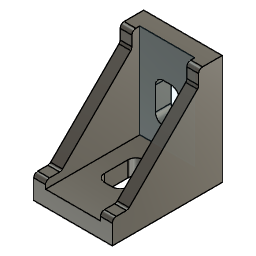
angle_bracket (Autodesk Fusion 360 design; units mm, degrees)
Autodesk Fusion 360 part; units mm, degrees
sketch "Sketch1" plane through (0, 0, 0) normal (1, 0, 0) x (0, 1, 0)
  line L0 (0, 0) -> (28, 0)
  line L1 (28, 0) -> (28, 28)
  line L2 (28, 28) -> (22, 28)
  line L3 (22, 28) -> (22, 24)
  line L4 (0, 0) -> (0, 6)
  line L5 (0, 6) -> (4, 6)
  line L6 (4, 6) -> (22, 24)
  dimension "d1" = 28
  dimension "d2" = 28
  constraint coincident L0.start L4.start
  constraint horizontal L0
  constraint perpendicular L0 L1
  constraint perpendicular L1 L2
  constraint perpendicular L2 L3
  constraint perpendicular L0 L4
  constraint perpendicular L4 L5
  measures "d1" distance of L0.start L0.end
  measures "d2" distance of L0.end L1.end
extrude "Extrude1" add sketch "Sketch1" along normal blind 3
sketch "Sketch2" plane through (3, 0, 0) normal (1, 0, 0) x (0, 1, 0)
  line L0 (0, 0) -> (28, 0)
  line L1 (28, 0) -> (28, 28)
  line L2 (28, 28) -> (22, 28)
  line L3 (22, 28) -> (22, 24)
  line L4 (22, 24) -> (4, 6)
  line L5 (4, 6) -> (0, 6)
  line L6 (0, 6) -> (0, 0)
  line L7 (0, 0) -> (28, 0)
  line L8 (28, 0) -> (28, 4)
  line L9 (24, 4) -> (0, 4)
  line L10 (0, 4) -> (0, 0)
  line L11 (28, 28) -> (24, 28)
  line L12 (24, 28) -> (24, 4)
  line L13 (24, 0) -> (28, 0)
  line L14 (28, 0) -> (28, 28)
  dimension "d5" = 4
  dimension "d6" = 28
  constraint horizontal L7
  constraint vertical L8
  constraint horizontal L9
  constraint vertical L10
  constraint coincident L1 L8.end
  constraint coincident L0.start L6.end
  constraint horizontal L11
  constraint vertical L12
  constraint horizontal L13
  constraint vertical L14
  constraint coincident L1.end L2.start
  measures "d5" distance of L1.end L11.end
  measures "d6" distance of L1.end L0.end
extrude "Extrude2" add sketch "Sketch2" along normal blind 14 contours L0 L1 L2 L6 L7 L8 L9 L10 L11 L12 L13 L14
sketch "Sketch3" plane through (17, 0, 0) normal (1, 0, 0) x (0, 1, 0)
  line L0 (28, 0) -> (28, 28)
  line L1 (28, 28) -> (24, 28)
  line L2 (24, 28) -> (24, 4)
  line L3 (24, 4) -> (0, 4)
  line L4 (0, 4) -> (0, 0)
  line L5 (0, 0) -> (28, 0)
  line L6 (0, 0) -> (28, 0)
  line L7 (28, 28) -> (28, 0)
  line L8 (28, 28) -> (22, 28)
  line L9 (22, 28) -> (22, 24)
  line L10 (22, 24) -> (4, 6)
  line L11 (4, 6) -> (0, 6)
  line L12 (0, 6) -> (0, 0)
  constraint coincident L4.end L5.start
  constraint coincident L0.start L5.end
  constraint coincident L0.end L1.start
  constraint perpendicular L2 L8
  constraint perpendicular L8 L9
  constraint perpendicular L9 L11
  constraint perpendicular L6 L12
sketch "Sketch4" plane through (17, 0, 0) normal (1, 0, 0) x (0, 1, 0)
extrude "Extrude3" add sketch "Sketch3" along normal blind 3
sketch "Sketch5" plane through (0, 24, 0) normal (0, -1, 0) x (1, 0, 0)
  line L0 (3, 28) -> (3, 4)
  line L1 (3, 4) -> (17, 4)
  line L2 (17, 4) -> (17, 28)
  line L3 (17, 28) -> (3, 28)
fillet "Fillet1" radius 1 1 edges at (1.5, 22, 28)
fillet "Fillet2" radius 1 1 edges at (18.5, 22, 28)
fillet "Fillet3" radius 1 1 edges at (1.5, 0, 6)
fillet "Fillet4" radius 1 1 edges at (18.5, 0, 6)
fillet "Fillet5" radius 1 1 edges at (1.5, 4, 6)
fillet "Fillet6" radius 1 1 edges at (18.5, 4, 6)
fillet "Fillet7" radius 1 1 edges at (1.5, 22, 24)
fillet "Fillet8" radius 1 1 edges at (18.5, 22, 24)
sketch "Sketch6" plane through (0, 24, 0) normal (0, -1, 0) x (1, 0, 0)
  line L0 (11, 19) -> (9, 19)
  line L1 (7, 17) -> (7, 11)
  line L2 (9, 9) -> (11, 9)
  line L3 (13, 11) -> (13, 17)
  line L4 (13, 19) -> (7, 9) construction
  line L5 (7, 19) -> (13, 9) construction
  arc A0 (9, 19) -> (7, 17) centre (9, 17) ccw
  arc A1 (13, 17) -> (11, 19) centre (11, 17) ccw
  arc A2 (11, 9) -> (13, 11) centre (11, 11) ccw
  arc A3 (7, 11) -> (9, 9) centre (9, 11) ccw
  point P0 (10, 14)
  dimension "d27" = 6
  dimension "d28" = 10
  dimension "d29" = 2
  constraint horizontal L0
  constraint perpendicular L0 L1
  constraint parallel L0 L2
  constraint parallel L1 L3
  constraint coincident L4 P0
  constraint coincident L5 P0
  constraint coincident L5.start L0
  constraint coincident L5.start L1
  constraint tangent L0 A0
  constraint tangent L1 A0
  constraint coincident L4.start L3
  constraint coincident L4.start L0
  constraint tangent L3 A1
  constraint tangent L0 A1
  constraint equal A0 A1
  constraint coincident L5.end L3
  constraint coincident L5.end L2
  constraint tangent L3 A2
  constraint tangent L2 A2
  constraint equal A0 A2
  constraint coincident L4.end L1
  constraint coincident L4.end L2
  constraint tangent L1 A3
  constraint tangent L2 A3
  constraint equal A0 A3
  measures "d27" distance of L4.end L5.end
  measures "d28" distance of L5.start L4.end
  measures "d29" radius of A0
extrude "Extrude4" cut sketch "Sketch6" against normal blind 7
sketch "Sketch7" plane through (0, 0, 4) normal (0, 0, 1) x (-1, 0, 0)
  line L0 (-3, -24) -> (-3, 0)
  line L1 (-3, 0) -> (-17, 0)
  line L2 (-17, 0) -> (-17, -24)
  line L3 (-17, -24) -> (-3, -24)
  line L4 (-9, -9) -> (-11, -9)
  line L5 (-13, -11) -> (-13, -17)
  line L6 (-11, -19) -> (-9, -19)
  line L7 (-7, -17) -> (-7, -11)
  line L8 (-7, -9) -> (-13, -19) construction
  line L9 (-13, -9) -> (-7, -19) construction
  arc A0 (-9, -19) -> (-7, -17) centre (-9, -17) ccw
  arc A1 (-7, -11) -> (-9, -9) centre (-9, -11) ccw
  arc A2 (-13, -17) -> (-11, -19) centre (-11, -17) ccw
  arc A3 (-11, -9) -> (-13, -11) centre (-11, -11) ccw
  point P0 (-10, -14)
  dimension "d32" = 6
  dimension "d33" = 10
  dimension "d34" = 2
  constraint horizontal L4
  constraint perpendicular L4 L5
  constraint parallel L4 L6
  constraint parallel L5 L7
  constraint coincident L8 P0
  constraint coincident L9 P0
  constraint coincident L9.end L6
  constraint coincident L9.end L7
  constraint tangent L6 A0
  constraint tangent L7 A0
  constraint coincident L8.start L4
  constraint coincident L8.start L7
  constraint tangent L4 A1
  constraint tangent L7 A1
  constraint equal A0 A1
  constraint coincident L8.end L6
  constraint coincident L8.end L5
  constraint tangent L6 A2
  constraint tangent L5 A2
  constraint equal A0 A2
  constraint coincident L9.start L5
  constraint coincident L9.start L4
  constraint tangent L5 A3
  constraint tangent L4 A3
  constraint equal A0 A3
  measures "d32" distance of L8.end L9.end
  measures "d33" distance of L9.start L8.end
  measures "d34" radius of A0
extrude "Extrude5" cut sketch "Sketch7" against normal blind 4 contours L4 L5 L6 L7 A0 A1 A2 A3
